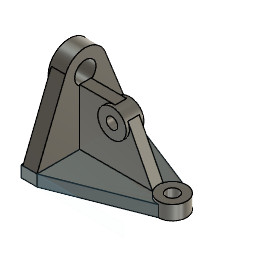
MARS 5 (Autodesk Fusion 360 design; units mm, degrees)
part number: 2026-05-31-20-59-38-534
Autodesk Fusion 360 part; units mm, degrees
note: some values were not read from the file. Set by a fixed rule: which sketch regions a step uses.
sketch "Sketch1" plane through (0, 0, 0) normal (0, 0, 1) x (1, 0, 0)
  line L0 (72.5, 68) -> (-72.5, 68)
  line L1 (-72.5, 68) -> (-72.5, -68)
  line L2 (-72.5, -68) -> (72.5, -68)
  line L3 (72.5, -68) -> (72.5, 68)
  line L4 (72.5, 68) -> (-72.5, -68) construction
  line L5 (-72.5, 68) -> (72.5, -68) construction
  dimension "d2" = 145
  dimension "d3" = 136
  constraint horizontal L0
  constraint perpendicular L0 L1
  constraint parallel L0 L2
  constraint parallel L1 L3
  constraint coincident L4 origin
  constraint coincident L5 origin
  measures "d2" distance of L1.end L2.end
  measures "d3" distance of L0.end L1.end
extrude "Extrude1" add sketch "Sketch1" along normal blind 136 makes body 1
sketch "Sketch2" plane through (0, -68, 0) normal (0, -1, 0) x (1, 0, 0)
  line L0 (-72.5, 0) -> (72.5, 0)
  line L1 (72.5, 0) -> (72.5, 136)
  line L2 (72.5, 136) -> (-72.5, 136)
  line L3 (-72.5, 136) -> (-72.5, 0)
  line L4 (-72.5, 136) -> (-50, 136)
  line L5 (-50, 136) -> (-50, 16)
  line L6 (-50, 16) -> (72.5, 16)
  line L7 (72.5, 0) -> (-72.5, 0)
  line L8 (72.5, 16) -> (72.5, 0)
  line L9 (-72.5, 0) -> (-72.5, 136)
  dimension "d6" = 136
  dimension "d7" = 16
  constraint coincident L2.end L3.start
  constraint coincident L2 L4.end
  constraint perpendicular L4 L5
  constraint coincident L1 L6.end
  constraint perpendicular L1 L6
  constraint coincident L0.end L1.start
  constraint coincident L0.start L3.end
  measures "d6" distance of L0.start L2.end
  measures "d7" distance of L6.end L0.end
extrude "Extrude2" cut sketch "Sketch2" against normal blind 290 contours L1 L2 L5 L6 bodies 1
sketch "Sketch3" plane through (-50, 0, 0) normal (1, 0, 0) x (0, 1, 0)
  line L0 (68, 16) -> (68, 136)
  line L1 (68, 136) -> (-68, 136)
  line L2 (-68, 136) -> (-68, 16)
  line L3 (-68, 16) -> (68, 16)
  line L4 (-68, 109.876) -> (68, 109.876) construction
  line L5 (0, 136) -> (0, 16) construction
  circle A0 centre (0, 109.876) radius 30
  circle A1 centre (0, 109.876) radius 15
  line L6 (-30, 109.876) -> (-68, 16)
  line L7 (30, 109.876) -> (68, 16)
  dimension "d10" = 60
  dimension "d11" = 30
  constraint coincident L2 L4.start
  constraint coincident L0 L4.end
  constraint perpendicular L0 L4
  constraint midpoint L1 L5.start
  constraint midpoint L3 L5.end
  constraint midpoint L4 A0.centre
  constraint concentric A0 A1
  constraint coincident A0 L6.start
  constraint coincident L4 L6.start
  constraint coincident L2.end L3.start
  constraint coincident L4 L7.start
  constraint coincident A0 L7.start
  constraint coincident L0.start L3.end
  measures "d10" diameter of A0
  measures "d11" diameter of A1
extrude "Extrude3" cut sketch "Sketch3" against normal blind 50 contours L0 L1 A0 L7 | L1 L2 A0 L6 bodies 1
sketch "Sketch4" plane through (-50, 0, 0) normal (1, 0, 0) x (0, 1, 0)
  arc A0 (-14.7492, 136) -> (-30, 109.876) centre (0, 109.876) ccw
  line L0 (-30, 109.876) -> (-68, 16)
  line L1 (-68, 16) -> (68, 16)
  line L2 (68, 16) -> (30, 109.876)
  arc A1 (30, 109.876) -> (14.7492, 136) centre (0, 109.876) ccw
  line L3 (14.7492, 136) -> (-14.7492, 136)
  line L4 (-20, 106) -> (20, 106) construction
  circle A2 centre (0, 106) radius 15
  circle A3 centre (0, 106) radius 30
  point P0 (-68, 0)
  dimension "d14" = 106
  dimension "d15" = 30
  dimension "d16" = 60
  constraint horizontal L4
  constraint midpoint L4 A2.centre
  constraint concentric A2 A3
  measures "d14" vertical distance of L4.start P0
  measures "d15" diameter of A2
  measures "d16" diameter of A3
extrude "Extrude4" cut sketch "Sketch4" against normal blind 50 contours A2 bodies 1
sketch "Sketch5" plane through (-50, 0, 0) normal (1, 0, 0) x (0, 1, 0)
  circle A0 centre (0, 106) radius 15
  arc A1 (-14.7492, 136) -> (-30, 109.876) centre (0, 109.876) ccw
  line L0 (-30, 109.876) -> (-68, 16)
  line L1 (-68, 16) -> (68, 16)
  line L2 (68, 16) -> (30, 109.876)
  arc A2 (30, 109.876) -> (14.7492, 136) centre (0, 109.876) ccw
  line L3 (14.7492, 136) -> (-14.7492, 136)
  circle A3 centre (0, 106) radius 30
  dimension "d19" = 60
  constraint concentric A0 A3
  measures "d19" diameter of A3
extrude "Extrude5" cut sketch "Sketch5" against normal blind 120 contours A1 L0 L1 L2 A2 L3 bodies 1 makes body 2 at (-57.5, 29.8509, 103.013)
sketch "Sketch6" plane through (-50, 0, 0) normal (1, 0, 0) x (0, 1, 0)
  circle A0 centre (0, 106) radius 30
  circle A1 centre (0, 106) radius 15
  line L0 (68, 16) -> (27.8838, 117.0677)
  line L1 (0, 0) -> (0, 136) construction
  line L2 (68, 16) -> (27.8838, 117.0677)
  line L3 (-68, 16) -> (-27.8838, 117.0677)
  line L4 (-68, 16) -> (68, 16)
  constraint coincident A0 L0.end
  constraint tangent A0 L0
  constraint coincident L1.start origin
  constraint coincident A0 L1.end
  constraint vertical L1
  constraint symmetric L2.start L0 L4.end
  constraint symmetric L2.end L0 L0.end
  constraint coincident A0 L3.end
  constraint tangent A0 L3
extrude "Extrude6" add sketch "Sketch6" against normal blind 20 contours A0 L0 L2 L3 L4 bodies 1 2
sketch "Sketch7" plane through (0, -68, 0) normal (0, -1, 0) x (1, 0, 0)
  line L0 (72.5, 16) -> (-50, 16)
  line L1 (-50, 16) -> (-70, 16)
  line L2 (-70, 16) -> (-72.5, 16)
  line L3 (-72.5, 16) -> (-72.5, 0)
  line L4 (-72.5, 0) -> (72.5, 0)
  line L5 (72.5, 0) -> (72.5, 16)
sketch "Sketch8" plane through (0, 0, 16) normal (0, 0, 1) x (-1, 0, 0)
  line L0 (50, -68) -> (50, 68)
  line L1 (50, 68) -> (-72.5, 68)
  line L2 (-72.5, 68) -> (-72.5, -68)
  line L3 (-72.5, -68) -> (50, -68)
  line L4 (50, 0) -> (-72.5, 0) construction
  circle A0 centre (-72.5, 0) radius 9
  circle A1 centre (-72.5, 0) radius 20
  dimension "d24" = 18
  dimension "d25" = 40
  constraint midpoint L0 L4.start
  constraint midpoint L2 L4.end
  constraint coincident L4.end A0.centre
  measures "d24" diameter of A0
  measures "d25" diameter of A1
extrude "Extrude7" add sketch "Sketch8" along normal blind 25 contours L2 A0 A1 | L2 A0 A1 bodies 1
sketch "Sketch9" plane through (0, 0, 16) normal (0, 0, 1) x (-1, 0, 0)
  arc A0 (-72.5, -20) -> (-72.5, 20) centre (-72.5, 0) ccw
  line L0 (-72.5, -20) -> (-72.5, -68)
  line L1 (-72.5, -68) -> (50, -68)
  line L2 (50, -68) -> (50, 68)
  line L3 (50, 68) -> (-72.5, 68)
  line L4 (-72.5, 68) -> (-72.5, 20)
  line L5 (-72.5, -20) -> (50, -68)
  line L6 (50, -68) -> (-72.5, -68)
  line L7 (-72.5, -20) -> (-72.5, -68)
  constraint coincident A0.start L0.start
  constraint coincident L1.end L2.start
  constraint coincident L0.end L1.start
extrude "Extrude8" cut sketch "Sketch9" against normal blind 40 contours L0 L1 L5 L6 L7 bodies 1
sketch "Sketch10" plane through (0, 0, 16) normal (0, 0, 1) x (-1, 0, 0)
  line L0 (-72.5, -20) -> (50, -68)
  line L1 (50, -68) -> (50, 68)
  line L2 (50, 68) -> (-72.5, 68)
  line L3 (-72.5, 68) -> (-72.5, 20)
  arc A0 (-72.5, -20) -> (-72.5, 20) centre (-72.5, 0) ccw
  line L4 (-72.5, 20) -> (50, 68)
  line L5 (50, 68) -> (-72.5, 68)
  line L6 (-72.5, 68) -> (-72.5, 20)
  constraint coincident L3.end A0.end
  constraint coincident L1.end L2.start
  constraint coincident L2.end L3.start
extrude "Extrude9" cut sketch "Sketch10" against normal blind 50 contours L2 L3 L4 L5 L6 bodies 1
sketch "Sketch11" plane through (16.4434, -41.965, 0) normal (0.364829, -0.931074, 0) x (0.931074, 0.364829, 0)
  line L0 (-71.3621, 0) -> (60.2063, 0)
  line L1 (60.2063, 0) -> (60.2063, 16)
  line L2 (60.2063, 16) -> (-71.3621, 16)
  line L3 (-71.3621, 16) -> (-71.3621, 0)
extrude "Extrude10" cut 1 faces at (69.1036, -0.4575, 16) along direction (0, 0, -1) blind 40 on bodies 1 bodies 1
extrude "Extrude11" cut 1 faces at (56.2746, 1.4407, 41) along direction (0, 0, -1) blind 50 on bodies 1 bodies 1
sketch "Sketch12" plane through (0, 0, 16) normal (0, 0, 1) x (-1, 0, 0)
  line L0 (50, 68) -> (-72.5, 20)
  arc A0 (-72.5, -20) -> (-72.5, 20) centre (-72.5, 0) ccw
  line L1 (-72.5, -20) -> (50, -68)
  line L2 (50, -68) -> (50, 68)
sketch "Sketch13" plane through (0, 0, 0) normal (0, 0, -1) x (1, 0, 0)
  arc A0 (72.5, 20) -> (72.5, -20) centre (72.5, 0) ccw
  line L0 (72.5, 20) -> (-50, 68)
  line L1 (-50, 68) -> (-72.5, 68)
  line L2 (-72.5, 68) -> (-72.5, -68)
  line L3 (-72.5, -68) -> (-50, -68)
  line L4 (-50, -68) -> (72.5, -20)
  circle A1 centre (72.5, 0) radius 9
  circle A2 centre (72.5, 0) radius 20
  dimension "d37" = 18
  dimension "d38" = 40
  constraint concentric A0 A1
  constraint concentric A0 A2
  measures "d37" diameter of A1
  measures "d38" diameter of A2
extrude "Extrude12" add sketch "Sketch13" against normal blind 20 contours A0 A2 bodies 1
sketch "Sketch14" plane through (0, 0, 0) normal (0, 1, 0) x (1, 0, 0)
  line L0 (0, 0) -> (0, -61) construction
  line L1 (0, -61) -> (-75, -61) construction
  circle A0 centre (0, -75) radius 8
  circle A1 centre (0, -75) radius 20
  dimension "d43" = 61
  dimension "d44" = 75
  dimension "d45" = 16
  dimension "d46" = 40
  constraint coincident L0.start origin
  constraint vertical L0
  constraint perpendicular L0 L1
  constraint concentric A0 A1
  measures "d43" distance of L0.start L0.end
  measures "d44" distance of L0.end L1.end
  measures "d45" diameter of A0
  measures "d46" diameter of A1
extrude "Extrude13" add sketch "Sketch14" along normal blind 12.5 and the other way blind 12.5 separate body makes body 3
sketch "Sketch15" plane through (0, -68, 0) normal (0, -1, 0) x (1, 0, 0)
sketch "Sketch16" plane through (0, 0, 0) normal (0, 1, 0) x (1, 0, 0)
  line L0 (0, -95) -> (-50, -95)
  line L1 (-50, -95) -> (-50, -16)
  line L2 (-50, -16) -> (52.5, -16)
  line L3 (52.5, -16) -> (17.821, -84.078)
  circle A0 centre (0, -75) radius 20
  constraint horizontal L0
  constraint perpendicular L0 L1
  constraint perpendicular L1 L2
  constraint tangent L3 A0
  constraint coincident L3.end A0
extrude "Extrude14" add sketch "Sketch16" along normal blind 8 and the other way blind 8 contours L0 L1 L2 L3 A0 bodies 1 3
